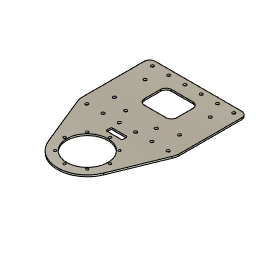
Trunk Side Plates v2 (Autodesk Fusion 360 design; units mm, degrees)
Autodesk Fusion 360 part; units mm, degrees
sketch "Sketch1" plane through (0, 0, 0) normal (0, 0, 1) x (1, 0, 0)
  line L0 (180, 133.6216) -> (180, 250)
  line L1 (170, 260) -> (10, 260)
  line L2 (0, 250) -> (0, 133.4829)
  circle A0 centre (90.016, 55) radius 38
  circle A1 centre (90.016, 55) radius 42 construction
  circle A2 centre (30, 165) radius 2.75
  circle A3 centre (30, 221.5) radius 2.75
  line L3 (2.627, 123.5637) -> (39.0941, 34.2163)
  line L4 (177.3504, 123.503) -> (140.9438, 34.2308)
  arc A4 (0, 133.4829) -> (2.627, 123.5637) centre (39.6611, 138.6792) ccw
  arc A5 (177.3504, 123.503) -> (180, 133.6216) centre (140.312, 138.6078) ccw
  arc A6 (10, 260) -> (0, 250) centre (10, 250) ccw
  arc A7 (180, 250) -> (170, 260) centre (170, 250) ccw
  arc A8 (39.0941, 34.2163) -> (140.9438, 34.2308) centre (90.016, 55) ccw
  circle A9 centre (90, 97) radius 2.25
  circle A10 centre (60.3062, 84.6872) radius 2.25
  circle A11 centre (48.016, 54.984) radius 2.25
  circle A12 centre (60.3288, 25.2902) radius 2.25
  circle A13 centre (90.032, 13) radius 2.25
  circle A14 centre (119.7258, 25.3128) radius 2.25
  circle A15 centre (132.016, 55.016) radius 2.25
  circle A16 centre (119.7032, 84.7098) radius 2.25
  circle A17 centre (150, 221.5) radius 2.75
  circle A18 centre (150, 165) radius 2.75
  circle A19 centre (61.75, 154) radius 2.75
  circle A20 centre (118.25, 154) radius 2.75
  line L5 (77.016, 104) -> (103.016, 104)
  line L6 (105.016, 106) -> (105.016, 112)
  line L7 (103.016, 114) -> (77.016, 114)
  line L8 (75.016, 112) -> (75.016, 106)
  arc A21 (77.016, 114) -> (75.016, 112) centre (77.016, 112) ccw
  arc A22 (75.016, 106) -> (77.016, 104) centre (77.016, 106) ccw
  arc A23 (103.016, 104) -> (105.016, 106) centre (103.016, 106) ccw
  arc A24 (105.016, 112) -> (103.016, 114) centre (103.016, 112) ccw
  circle A25 centre (15, 129) radius 2.75
  circle A26 centre (15, 250) radius 2.75
  circle A27 centre (45, 250) radius 2.75
  circle A28 centre (45, 129) radius 2.75
  circle A29 centre (75, 250) radius 2.75
  circle A30 centre (105, 250) radius 2.75
  circle A31 centre (135, 250) radius 2.75
  circle A32 centre (135, 129) radius 2.75
  circle A33 centre (165, 250) radius 2.75
  circle A34 centre (165, 129) radius 2.75
  line L9 (110, 180) -> (70, 180)
  line L10 (60, 190) -> (60, 220)
  line L11 (70, 230) -> (110, 230)
  line L12 (120, 220) -> (120, 190)
  arc A35 (70, 230) -> (60, 220) centre (70, 220) ccw
  arc A36 (120, 220) -> (110, 230) centre (110, 220) ccw
  arc A37 (110, 180) -> (120, 190) centre (110, 190) ccw
  arc A38 (60, 190) -> (70, 180) centre (70, 190) ccw
  circle A39 centre (75, 129) radius 2.75
  circle A40 centre (105, 129) radius 2.75
  point P0 (180, 260)
  point P1 (0, 260)
  point P2 (0, 130)
  point P3 (75.016, 104)
  point P4 (105.016, 114)
  point P5 (75.016, 114)
  dimension "d1" = 260
  dimension "d3" = 76
  dimension "d4" = 84
  dimension "d5" = 110
  dimension "d8" = 130
  dimension "d9" = 180
  dimension "d10" = 40
  dimension "d11" = 10
  dimension "d12" = 4.5
  dimension "d13" = 90
  dimension "d15" = 360
  dimension "d16" = 5.5
  dimension "d17" = 5.5
  dimension "d18" = 56.5
  dimension "d19" = 110
  dimension "d22" = 120
  dimension "d23" = 0
  dimension "d24" = 30
  dimension "d25" = 30
  dimension "d26" = 5.5
  dimension "d27" = 5.5
  dimension "d28" = 56.5
  dimension "d29" = 61.75
  dimension "d32" = 30
  dimension "d33" = 10
  dimension "d34" = 15
  dimension "d35" = 49
  dimension "d36" = 2
  dimension "d37" = 5.5
  dimension "d38" = 15
  dimension "d39" = 5.5
  dimension "d40" = 15
  dimension "d41" = 10
  dimension "d44" = 30
  dimension "d45" = 0
  dimension "d46" = 60
  dimension "d47" = 60
  dimension "d48" = 50
  dimension "d49" = 30
  dimension "d50" = 10
  dimension "d54" = 40
  dimension "d57" = 15
  dimension "d60" = 60
  dimension "d61" = 0
  constraint vertical L0
  constraint horizontal L1
  constraint vertical L2
  constraint concentric A0 A1
  constraint concentric A1 A8
  constraint tangent L4 A8
  constraint tangent L3 A8
  constraint coincident P2 L3
  constraint coincident L2 P2
  constraint tangent L3 A4
  constraint tangent L4 A5
  constraint equal A4 A5
  constraint coincident P1 L1
  constraint coincident P1 L2
  constraint tangent L1 A6
  constraint tangent L2 A6
  constraint coincident P0 L0
  constraint coincident P0 L1
  constraint tangent L0 A7
  constraint tangent L1 A7
  constraint equal A6 A7
  constraint coincident A1 A9.centre
  constraint horizontal L5
  constraint vertical L6
  constraint horizontal L7
  constraint vertical L8
  constraint coincident P5 L7
  constraint coincident P5 L8
  constraint tangent L7 A21
  constraint tangent L8 A21
  constraint coincident P3 L5
  constraint coincident P3 L8
  constraint tangent L5 A22
  constraint tangent L8 A22
  constraint equal A21 A22
  constraint tangent L5 A23
  constraint tangent L6 A23
  constraint equal A21 A23
  constraint coincident P4 L6
  constraint coincident P4 L7
  constraint tangent L6 A24
  constraint tangent L7 A24
  constraint equal A21 A24
  constraint horizontal L9
  constraint vertical L10
  constraint horizontal L11
  constraint vertical L12
  constraint tangent L10 A35
  constraint tangent L11 A35
  constraint tangent L11 A36
  constraint tangent L12 A36
  constraint equal A35 A36
  constraint tangent L9 A37
  constraint tangent L12 A37
  constraint equal A35 A37
  constraint tangent L9 A38
  constraint tangent L10 A38
  constraint equal A35 A38
  measures "d1" distance of origin P1
  measures "d3" diameter of A0
  measures "d4" diameter of A1
  measures "d5" diameter of A8
  measures "d8" distance of origin P2
  measures "d9" distance of P0 P1
  measures "d10" radius of A4
  measures "d11" radius of A6
  measures "d12" diameter of A9
  measures "d13" distance of L2 A9.centre
  measures "d16" diameter of A2
  measures "d17" diameter of A3
  measures "d18" distance of A2.centre A3.centre
  measures "d19" vertical distance of A0.centre A2.centre
  measures "d24" horizontal distance of origin A2.centre
  measures "d25" horizontal distance of origin A3.centre
  measures "d26" diameter of A19
  measures "d27" diameter of A20
  measures "d28" distance of A19.centre A20.centre
  measures "d29" distance of L2 A19.centre
  measures "d32" distance of P4 P5
  measures "d33" distance of P3 P5
  measures "d34" horizontal distance of A0.centre P3
  measures "d35" distance of A0.centre L5
  measures "d36" radius of A21
  measures "d37" diameter of A25
  measures "d38" distance of L2 A25.centre
  measures "d39" diameter of A26
  measures "d40" distance of L2 A26.centre
  measures "d41" distance of L1 A26.centre
  measures "d46" distance of L2 L10
  measures "d47" distance of L0 L12
  measures "d48" distance of L9 L11
  measures "d49" distance of L1 L11
  measures "d50" radius of A35
  measures "d54" distance of A20.centre L7
  measures "d57" distance of L7 A28.centre
extrude "Extrude1" add sketch "Sketch1" along normal blind 3 contours L0 L1 L2 L3 L4 A4 A5 A6 A7 A8 | A39 | A40
extrude "Extrude3" cut sketch "Sketch1" along normal through all contours A39 | A40
extrude "Extrude2" [suppressed]
equation "d29 = ( ( 180 - 56.5 ) / 2 ) * 1 mm"
